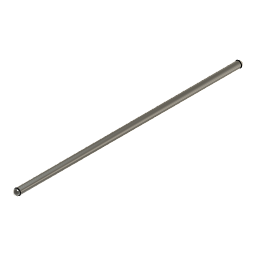
Schiebemechanismus Stab (Autodesk Fusion 360 design; units mm, degrees)
Autodesk Fusion 360 part; units mm, degrees
sketch "Skizze1" plane through (0, 0, 0) normal (0, 1, 0) x (1, 0, 0)
  circle A0 centre (0, 0) radius 4
  dimension "d1" = 8
  constraint coincident A0.centre origin
  measures "d1" diameter of A0
extrude "Extrusion1" add sketch "Skizze1" along normal blind 300
fillet "Abrundung1" radius 4 1 edges at (-3.7293, 0, 1.4465)
fillet "Abrundung2" radius 4 1 edges at (-3.7293, 300, 1.4465)
